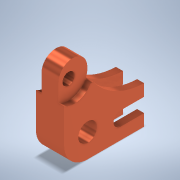
# Autodesk Inventor part: FIGURA3_U3_MINIPROYECTO
Saved by Autodesk Inventor 2021 (Build 250183000, 183)
## iProperties
Created: 2021-02-09
Part Number: FIGURA3_U3_MINIPROYECTO
Material: Generic
Document SubType Name: Modeling
Designer: aby_2
Density: 1 g/cm^3
Appearance: Generic
Author: aby_2
Autodesk Inventor part; units mm, degrees
ref_plane "YZ Plane" through (0, 0, 0) normal (1, 0, 0) x (0, 1, 0)
ref_plane "XZ Plane" through (0, 0, 0) normal (0, 1, 0) x (-1, 0, 0)
ref_plane "XY Plane" through (0, 0, 0) normal (0, 0, 1) x (1, 0, 0)
sketch "Sketch1" plane through (0, 0, 0) normal (0, 1, 0) x (-1, 0, 0)
  line L0 (0, 42.5) -> (0, -42.5)
  line L1 (15, 0) -> (-15, 0)
  line L2 (0, 42.5) -> (15, 42.5)
  line L3 (15, 42.5) -> (15, -42.5)
  line L4 (15, -42.5) -> (-15, -42.5)
  line L5 (0, 42.5) -> (-15, 42.5)
  line L6 (-15, 42.5) -> (-15, -42.5)
  point P0 (0, 0)
  point P1 (0, 0)
  point P2 (0, 0)
  constraints: 14 end point, 4 horizontal, 3 perpendicular, 2 coincident, 2 midpoint, 2 vertical
extrude "Extrusion1" add sketch "Sketch1" along normal blind 95
fillet "Fillet1" radius 25 1 edges at (-7.5, 0, 42.5)
sketch "Sketch2" plane through (15, 0, -42.5) normal (1, 0, 0) x (0, 0, -1)
  arc A0 (-85, 25) -> (-60, 0) centre (-60, 25) ccw projected
  line L0 (-60, 0) -> (0, 0) projected
  line L1 (0, 0) -> (0, 95) projected
  line L2 (-85, 95) -> (0, 95) projected
  line L3 (-85, 25) -> (-85, 95) projected
  circle A1 centre (-60, 25) radius 10
  line L4 (0, 0) -> (0, 12.5)
  line L5 (0, 0) -> (0, 95) projected
  line L6 (0, 12.5) -> (-25, 12.5)
  line L7 (0, 12.5) -> (0, 27.5)
  line L8 (0, 27.5) -> (0, 40)
  line L9 (0, 40) -> (-40, 40)
  line L10 (0, 27.5) -> (-25, 27.5)
  arc A2 (-25, 27.5) -> (-25, 12.5) centre (-25, 20) ccw
  point P0 (-42.5, 0)
  dimension "d5" = 20
  dimension "d6" = 12.5
  dimension "d7" = 25
  dimension "d8" = 15
  dimension "d9" = 12.5
  dimension "d10" = 40
  constraints: 12 end point, 3 point on line, 2 centre point, 2 perpendicular, 2 point on circle, 1 coincident, 1 horizontal
  measures "d5" diameter of A1
  measures "d6" distance of L0.end L4.end
  measures "d7" distance of L4.end L6.end
  measures "d8" distance of L4.end L7.end
  measures "d9" distance of L7.end L8.end
  measures "d10" distance of L8.end L9.end
extrude "Extrusion2" cut sketch "Sketch2" against normal up to next contours L6 A2 L10 L1 | A1
sketch "Sketch3" plane through (15, 95, 42.5) normal (1, 0, 0) x (0, 0, -1)
  line L0 (85, -82.5) -> (60, -82.5) projected
  arc A0 (60, -67.5) -> (60, -82.5) centre (60, -75) ccw projected
  line L1 (60, -67.5) -> (85, -67.5) projected
  line L2 (85, -67.5) -> (85, 0) projected
  line L3 (0, 0) -> (85, 0) projected
  line L4 (0, -70) -> (0, 0) projected
  arc A1 (0, -70) -> (25, -95) centre (25, -70) ccw projected
  line L5 (25, -95) -> (85, -95) projected
  line L6 (85, -95) -> (85, -82.5) projected
  circle A2 centre (25, -70) radius 10 projected
  line L7 (25, -70) -> (25, 29)
  line L8 (25, -70) -> (-1.9532, 30.5909)
  line L9 (25, -70) -> (10.765, -16.8741)
  circle A3 centre (10.765, -16.8741) radius 6.5
  circle A4 centre (10.765, -16.8741) radius 20
  line L10 (0, 0) -> (85, 0) projected
  line L11 (85, 0) -> (0, 0) projected
  point P0 (42.5, -95)
  dimension "d13" = 15
  dimension "d14" = 55
  dimension "d15" = 13
  dimension "d17" = 40
  constraints: 6 end point, 2 centre point, 1 coincident, 1 point on line, 1 vertical
  measures "d13" angle of L7 L8
  measures "d14" distance of L7.start L9.end
  measures "d15" diameter of A3
  measures "d17" diameter of A4
extrude "Extrusion3" cut sketch "Sketch3" against normal up to next contours A3 L8 | L8 A3
extrude "Extrusion4" cut sketch "Sketch3" against normal blind 6 contours A4 L4 | L4 A4 L3 L8 A3 | L8 A3 L3 A4 L7 | L3 L8 A4 | A4 L7 | A4 L8 L3
fillet "Fillet2" radius 15 1 edges at (0, 95, 42.5)
sketch "Sketch5" plane through (15, 0, -42.5) normal (0, 0, -1) x (-1, 0, 0)
  line L0 (30, 12.5) -> (0, 12.5) projected
  line L1 (0, 0) -> (0, 12.5) projected
  line L2 (0, 0) -> (30, 0) projected
  line L3 (30, 0) -> (30, 12.5) projected
  line L4 (0, 0) -> (7.5, 0)
  line L5 (7.5, 0) -> (7.5, 40)
  line L6 (7.5, 40) -> (22.5, 40)
  line L7 (22.5, 40) -> (22.5, 0)
  point P0 (15, 0)
  dimension "d28" = 7.5
  dimension "d29" = 40
  dimension "d30" = 15
  constraints: 8 end point, 3 perpendicular, 2 point on line
  measures "d28" distance of L1.start L4.end
  measures "d29" distance of L4.end L5.end
  measures "d30" distance of L5.end L6.end
extrude "Extrusion6" cut sketch "Sketch5" against normal blind 40 contours L7 L2 L5 L0 | L0 L5 L6 L7
sketch "Sketch6" plane through (15, 0, 17.5) normal (1, 0, 0) x (0, 0, -1)
  arc A0 (-25, 61.2702) -> (-3.4989, 95) centre (-14.235, 78.1259) ccw projected
  line L0 (-25, 25) -> (-25, 61.2702) projected
  arc A1 (-25, 25) -> (0, 0) centre (0, 25) ccw projected
  line L1 (0, 0) -> (60, 0) projected
  line L2 (60, 0) -> (60, 12.5) projected
  line L3 (60, 12.5) -> (35, 12.5) projected
  arc A2 (35, 27.5) -> (35, 12.5) centre (35, 20) ccw projected
  line L4 (35, 27.5) -> (60, 27.5) projected
  line L5 (60, 27.5) -> (60, 95) projected
  line L6 (-3.4989, 95) -> (60, 95) projected
  circle A3 centre (0, 25) radius 10 projected
  line L7 (-14.235, 78.1259) -> (5.765, 78.1259)
  line L8 (60, 40) -> (60, 27.5) projected
  line L9 (60, 0) -> (60, 40)
  line L10 (60, 40) -> (20, 40) projected
  line L11 (60, 40) -> (20, 40)
  line L12 (20, 40) -> (20, 54)
  circle A4 centre (62, 110) radius 70
  point P0 (17.5, 0)
  point P1 (4.2372, 70.4594)
  point P2 (60, 40.0286)
  dimension "d33" = 140
  constraints: 8 end point, 2 collinear, 2 horizontal, 1 perpendicular, 1 point on circle, 3 other
extrude "Extrusion7" cut sketch "Sketch6" against normal up to next contours A0 L6 L5 A4
sketch "Sketch7" plane through (-15, 0, -42.5) normal (-1, 0, 0) x (0, 0, 1)
  circle A0 centre (60, 25) radius 10 projected
  circle A1 centre (74.235, 78.1259) radius 6.5 projected
  arc A2 (0, 40.0286) -> (55.7628, 70.4594) centre (-2, 110) ccw projected
  line L0 (0, 27.5) -> (0, 40.0286) projected
  line L1 (0, 27.5) -> (25, 27.5) projected
  arc A3 (25, 12.5) -> (25, 27.5) centre (25, 20) ccw projected
  line L2 (25, 12.5) -> (0, 12.5) projected
  line L3 (0, 0) -> (0, 12.5) projected
  line L4 (0, 0) -> (60, 0) projected
  arc A4 (60, 0) -> (85, 25) centre (60, 25) ccw projected
  line L5 (85, 25) -> (85, 80) projected
  arc A5 (85, 80) -> (70, 95) centre (70, 80) ccw projected
  line L6 (63.4989, 95) -> (70, 95) projected
  circle A6 centre (74.235, 78.1259) radius 20
  arc A7 (63.4989, 95) -> (55.7628, 70.4594) centre (74.235, 78.1259) ccw projected
  point P0 (42.5, 0)
  dimension "d36" = 40
  constraints: 1 centre point, 1 coincident
  measures "d36" diameter of A6
extrude "Extrusion8" cut sketch "Sketch7" against normal blind 6 contours A1 | A6 L6 A5 L5 | A6 L5 A5 L6
fillet "Fillet3" radius 15 1 edges at (0, 95, 20.9989)
sketch "Sketch8" plane through (-7.5, 40, -42.5) normal (0, -1, 0) x (1, 0, 0)
  line L0 (0, 0) -> (0, 40) projected
  line L1 (0, 40) -> (15, 40)
  line L2 (15, 0) -> (15, 40) projected
  line L3 (15, 40) -> (15, 0)
  line L4 (15, 0) -> (0, 0)
  line L5 (0, 0) -> (0, 40)
  point P0 (7.5, 42.5)
  constraints: 8 end point, 3 perpendicular, 1 horizontal
extrude "Extrusion9" cut sketch "Sketch8" against normal up to next
sketch "Sketch9" plane through (9, 95, 42.5) normal (1, 0, 0) x (0, 0, -1)
  circle A0 centre (25, -70) radius 10 projected
  arc A1 (29.2372, -24.5406) -> (85, -54.9714) centre (87, 15) ccw projected
  arc A2 (0, -33.7298) -> (29.2372, -24.5406) centre (10.765, -16.8741) ccw projected
  line L0 (0, -70) -> (0, -33.7298) projected
  arc A3 (0, -70) -> (25, -95) centre (25, -70) ccw projected
  line L1 (25, -95) -> (85, -95) projected
  line L2 (85, -95) -> (85, -82.5) projected
  line L3 (85, -82.5) -> (60, -82.5) projected
  arc A4 (60, -67.5) -> (60, -82.5) centre (60, -75) ccw projected
  line L4 (60, -67.5) -> (85, -67.5) projected
  line L5 (85, -67.5) -> (85, -54.9714) projected
  line L6 (10.765, -16.8741) -> (29.2372, -16.8741)
  circle A5 centre (29.2372, -16.8741) radius 10
  point P0 (42.5, -95)
  dimension "d42" = 20
  constraints: 2 end point, 1 centre point, 1 coincident, 1 horizontal
  measures "d42" diameter of A5
extrude "Extrusion10" cut sketch "Sketch9" along normal blind 10 contours A2 A5 A1 | A1 A5 A2
sketch "Sketch10" plane through (-9, 0, -42.5) normal (-1, 0, 0) x (0, 0, 1)
  circle A0 centre (74.235, 78.1259) radius 6.5 projected
  arc A1 (69.5996, 95) -> (55.6931, 85.6222) centre (69.5996, 80) ccw projected
  arc A2 (55.6931, 85.6222) -> (55.7628, 70.4594) centre (74.235, 78.1259) ccw projected
  arc A3 (55.7628, 70.4594) -> (85, 61.2702) centre (74.235, 78.1259) ccw projected
  line L0 (85, 80) -> (85, 61.2702) projected
  arc A4 (85, 80) -> (70, 95) centre (70, 80) ccw projected
  line L1 (69.5996, 95) -> (70, 95) projected
  line L2 (74.235, 78.1259) -> (42.5, 78.1259)
  circle A5 centre (54.235, 78.1259) radius 10
  point P0 (42.5, 0)
  dimension "d45" = 20
  constraints: 2 end point, 1 centre point, 1 horizontal, 1 point on circle, 1 point on line
  measures "d45" diameter of A5
extrude "Extrusion11" cut sketch "Sketch10" along normal blind 10 contours A5 A3 A2 L2 | L2 A2 A1 A5 | L2 A5 A1 A2 | A2 A3 A5 L2
body "Solid1"
